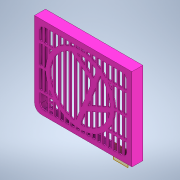
# Autodesk Inventor part: Rambo Case Lid
Saved by Autodesk Inventor 2023 (Build 270158000, 158)
## iProperties
Created: 2019-12-31
Part Number: Rambo Case Lid
Material: Generic
Document SubType Name: Modeling
Designer: pepd9
Density: 1 g/cm^3
Appearance: Default
Author: pepd9
Autodesk Inventor part; units mm, degrees
(part 1 of 2)
ref_plane "YZ Plane" through (0, 0, 0) normal (1, 0, 0) x (0, 1, 0)
ref_plane "XZ Plane" through (0, 0, 0) normal (0, 1, 0) x (-1, 0, 0)
sketch "Sketch1" plane through (0, 0, 0) normal (0, 0, 1) x (1, 0, 0)
  line L0 (3, 53.125) -> (3, 56.125)
  line L1 (3, 56.125) -> (137.52, 56.125)
  line L2 (143.52, 56.125) -> (143.52, 62.125)
  line L3 (143.52, 62.125) -> (-3, 62.125)
  line L4 (-3, 62.125) -> (-3, 53.125)
  line L5 (137.52, -56.125) -> (137.52, 56.125)
  line L6 (143.52, 56.125) -> (143.52, -56.125)
  line L7 (-3, 35.125) -> (-3, 53.125)
  line L8 (143.52, 62.125) -> (-3, 62.125)
  line L9 (-3, 62.125) -> (-3, 53.125)
  line L10 (3, 56.125) -> (33.535898, 56.125)
  line L11 (143.52, 56.125) -> (143.52, 62.125)
  line L12 (-3, 35.125) -> (-3, -52.125)
  arc A0 (-3, -52.125) -> (7, -62.125) centre (7, -52.125) ccw
  line L13 (7, -62.125) -> (143.52, -62.125)
  line L14 (143.52, -62.125) -> (143.52, -56.125)
  line L15 (137.52, -56.125) -> (8, -56.125)
  arc A1 (3, -51.125) -> (8, -56.125) centre (8, -51.125) ccw
  line L16 (3, -51.125) -> (3, 53.125)
  point P0 (0, 0)
  dimension "d0" = 6
  constraints: 34 end point, 4 point on circle, 2 centre point, 1 point on line
  measures "d0" distance between parallel lines of L6 L5
extrude "Extrusion1" add sketch "Sketch1" along normal blind 15
sketch "Sketch2" plane through (0, 0, 15) normal (0, 0, 1) x (1, 0, 0)
  line L0 (-3, 62.125) -> (-3, -52.125) projected
  arc A0 (-3, -52.125) -> (7, -62.125) centre (7, -52.125) ccw projected
  line L1 (7, -62.125) -> (143.52, -62.125) projected
  line L2 (143.52, -62.125) -> (143.52, 62.125) projected
  line L3 (143.52, 62.125) -> (-3, 62.125) projected
  point P0 (0, 0)
extrude "Extrusion2" add sketch "Sketch2" along normal blind 1.5
sketch "Sketch3" plane through (0, 0, 16.5) normal (0, 0, 1) x (1, 0, 0)
  line L0 (5, -47.125) -> (5, 47.125)
  line L1 (12, 54.125) -> (128.52, 54.125)
  line L2 (135.52, 47.125) -> (135.52, -47.125)
  line L3 (128.52, -54.125) -> (12, -54.125)
  arc A0 (5, -47.125) -> (12, -54.125) centre (12, -47.125) ccw
  arc A1 (128.52, -54.125) -> (135.52, -47.125) centre (128.52, -47.125) ccw
  arc A2 (135.52, 47.125) -> (128.52, 54.125) centre (128.52, 47.125) ccw
  arc A3 (12, 54.125) -> (5, 47.125) centre (12, 47.125) ccw
  line L4 (72.76, 54.125) -> (67.76, 54.125)
  line L5 (67.76, 54.125) -> (67.76, -54.125)
  line L6 (67.76, -54.125) -> (72.76, -54.125)
  line L7 (72.76, -54.125) -> (72.76, 54.125)
  line L8 (72.76, 54.125) -> (67.76, -54.125) construction
  line L9 (67.76, 54.125) -> (72.76, -54.125) construction
  line L10 (75.76, 54.125) -> (75.76, -54.125)
  line L11 (75.76, 54.125) -> (80.76, -54.125) construction
  line L12 (80.76, 54.125) -> (75.76, -54.125) construction
  line L13 (80.76, -54.125) -> (80.76, 54.125)
  line L14 (83.76, 54.125) -> (83.76, -54.125)
  line L15 (83.76, 54.125) -> (88.76, -54.125) construction
  line L16 (88.76, 54.125) -> (83.76, -54.125) construction
  line L17 (88.76, -54.125) -> (88.76, 54.125)
  line L18 (91.76, 54.125) -> (91.76, -54.125)
  line L19 (91.76, 54.125) -> (96.76, -54.125) construction
  line L20 (96.76, 54.125) -> (91.76, -54.125) construction
  line L21 (96.76, -54.125) -> (96.76, 54.125)
  line L22 (99.76, 54.125) -> (99.76, -54.125)
  line L23 (99.76, 54.125) -> (104.76, -54.125) construction
  line L24 (104.76, 54.125) -> (99.76, -54.125) construction
  line L25 (104.76, -54.125) -> (104.76, 54.125)
  line L26 (107.76, 54.125) -> (107.76, -54.125)
  line L27 (107.76, 54.125) -> (112.76, -54.125) construction
  line L28 (112.76, 54.125) -> (107.76, -54.125) construction
  line L29 (112.76, -54.125) -> (112.76, 54.125)
  line L30 (115.76, 54.125) -> (115.76, -54.125)
  line L31 (115.76, 54.125) -> (120.76, -54.125) construction
  line L32 (120.76, 54.125) -> (115.76, -54.125) construction
  line L33 (120.76, -54.125) -> (120.76, 54.125)
  line L34 (123.76, 54.125) -> (123.76, -54.125)
  line L35 (123.76, 54.125) -> (128.76, -54.125) construction
  line L36 (128.76, 54.125) -> (123.76, -54.125) construction
  line L37 (128.76, -54.125) -> (128.76, 54.125)
  line L38 (131.76, 54.125) -> (131.76, -54.125)
  line L39 (131.76, 54.125) -> (136.76, -54.125) construction
  line L40 (136.76, 54.125) -> (131.76, -54.125) construction
  line L41 (136.76, -54.125) -> (136.76, 54.125)
  line L42 (59.76, -54.125) -> (64.76, -54.125)
  line L43 (64.76, -54.125) -> (64.76, 54.125)
  line L44 (64.76, 54.125) -> (59.76, 54.125)
  line L45 (59.76, 54.125) -> (59.76, -54.125)
  line L46 (59.76, 54.125) -> (64.76, -54.125) construction
  line L47 (64.76, 54.125) -> (59.76, -54.125) construction
  line L48 (51.76, -54.125) -> (56.76, -54.125)
  line L49 (56.76, -54.125) -> (56.76, 54.125)
  line L50 (56.76, 54.125) -> (51.76, 54.125)
  line L51 (51.76, 54.125) -> (51.76, -54.125)
  line L52 (51.76, 54.125) -> (56.76, -54.125) construction
  line L53 (56.76, 54.125) -> (51.76, -54.125) construction
  line L54 (43.76, -54.125) -> (48.76, -54.125)
  line L55 (48.76, -54.125) -> (48.76, 54.125)
  line L56 (48.76, 54.125) -> (43.76, 54.125)
  line L57 (43.76, 54.125) -> (43.76, -54.125)
  line L58 (43.76, 54.125) -> (48.76, -54.125) construction
  line L59 (48.76, 54.125) -> (43.76, -54.125) construction
  line L60 (35.76, -54.125) -> (40.76, -54.125)
  line L61 (40.76, -54.125) -> (40.76, 54.125)
  line L62 (40.76, 54.125) -> (35.76, 54.125)
  line L63 (35.76, 54.125) -> (35.76, -54.125)
  line L64 (35.76, 54.125) -> (40.76, -54.125) construction
  line L65 (40.76, 54.125) -> (35.76, -54.125) construction
  line L66 (27.76, -54.125) -> (32.76, -54.125)
  line L67 (32.76, -54.125) -> (32.76, 54.125)
  line L68 (32.76, 54.125) -> (27.76, 54.125)
  line L69 (27.76, 54.125) -> (27.76, -54.125)
  line L70 (27.76, 54.125) -> (32.76, -54.125) construction
  line L71 (32.76, 54.125) -> (27.76, -54.125) construction
  line L72 (19.76, -54.125) -> (24.76, -54.125)
  line L73 (24.76, -54.125) -> (24.76, 54.125)
  line L74 (24.76, 54.125) -> (19.76, 54.125)
  line L75 (19.76, 54.125) -> (19.76, -54.125)
  line L76 (19.76, 54.125) -> (24.76, -54.125) construction
  line L77 (24.76, 54.125) -> (19.76, -54.125) construction
  line L78 (11.76, -54.125) -> (16.76, -54.125)
  line L79 (16.76, -54.125) -> (16.76, 54.125)
  line L80 (16.76, 54.125) -> (11.76, 54.125)
  line L81 (11.76, 54.125) -> (11.76, -54.125)
  line L82 (11.76, 54.125) -> (16.76, -54.125) construction
  line L83 (16.76, 54.125) -> (11.76, -54.125) construction
  line L84 (3.76, -54.125) -> (8.76, -54.125)
  line L85 (8.76, -54.125) -> (8.76, 54.125)
  line L86 (8.76, 54.125) -> (3.76, 54.125)
  line L87 (3.76, 54.125) -> (3.76, -54.125)
  line L88 (3.76, 54.125) -> (8.76, -54.125) construction
  line L89 (8.76, 54.125) -> (3.76, -54.125) construction
  line L90 (-3, 62.125) -> (-3, -52.125) projected
  arc A4 (-3, -52.125) -> (7, -62.125) centre (7, -52.125) ccw projected
  line L91 (7, -62.125) -> (143.52, -62.125) projected
  line L92 (143.52, -62.125) -> (143.52, 62.125) projected
  line L93 (143.52, 62.125) -> (-3, 62.125) projected
  point P0 (0, 0)
  point P1 (70.26, 0)
  point P2 (78.26, 0)
  point P3 (86.26, 0)
  point P4 (94.26, 0)
  point P5 (102.26, 0)
  point P6 (110.26, 0)
  point P7 (118.26, 0)
  point P8 (126.26, 0)
  point P9 (134.26, 0)
  point P10 (62.26, 0)
  point P11 (54.26, 0)
  point P12 (46.26, 0)
  point P13 (38.26, 0)
  point P14 (30.26, 0)
  point P15 (22.26, 0)
  point P16 (14.26, 0)
  point P17 (6.26, 0)
  point P18 (8.76, -53.33003)
  point P19 (8.76, 53.33003)
  point P20 (11.76, 54.120885)
  point P21 (11.76, -54.120885)
  point P22 (128.76, -54.120885)
  point P23 (128.76, 54.120885)
  point P24 (131.76, 53.33003)
  point P25 (131.76, -53.33003)
  dimension "d6" = 7
  dimension "d29" = 7
  dimension "d30" = 5
  dimension "d33" = 8
  dimension "d40" = 8
  constraints: 176 end point, 34 midpoint, 8 point on circle, 4 centre point, 4 tangent, 3 horizontal, 2 equal radius, 2 parallel, 1 collinear, 1 perpendicular, 170 other
  measures "d6" radius of A0
  measures "d29" radius of A1
  measures "d30" distance of L6.end L5.end
  measures "d33" distance of L4.end L10.start
  measures "d40" distance of L5.end L42.start
ref_plane "Work Plane1" through (-3, -62.125, 0) normal (0, 0, 1) x (1, 0, 0)
extrude "Extrusion4" cut sketch "Sketch3" against normal through all contours L0 A3 L85 A0 | L81 A3 L1 L79 L3 A0 | L75 L1 L73 L3 | L69 L1 L67 L3 | L63 L1 L61 L3 | L57 L1 L55 L3 | L51 L1 L49 L3 | L45 L1 L43 L3 | L5 L1 L7 L3 | L10 L1 L13 L3 | L14 L1 L17 L3 | L18 L1 L21 L3 | L22 L1 L25 L3 | L26 L1 L29 L3 | L30 L1 L33 L3 | L34 L1 A2 L37 A1 L3 | L38 A2 L2 A1
sketch "Sketch8" plane through (0, 0, 16.5) normal (0, 0, 1) x (1, 0, 0)
  circle A0 centre (65.9053, 0) radius 45
  line L0 (67.76, -54.125) -> (67.76, 54.125)
  line L1 (72.76, -54.125) -> (67.76, -54.125)
  circle A1 centre (65.9053, 0) radius 52
  line L2 (66.135277, -44.999412) -> (96.47099, 33.026332)
  line L3 (58.8415, -44.442128) -> (90.71627, 37.542186)
  line L4 (77.895632, -14.750892) -> (110.904226, -0.31086)
  line L5 (74.316291, -23.957225) -> (110.135552, -8.287631)
  line L6 (83.222966, 18.268842) -> (52.72419, 43.026252)
  line L7 (85.887401, 25.121972) -> (61.648183, 44.79818)
  point P0 (0, 0)
  point P1 (67.76, -44.961763)
  point P2 (67.76, -21.503073)
  point P3 (67.76, -40.820501)
  dimension "d56" = 90
  dimension "d58" = 54.125
  dimension "d59" = 7
  dimension "d60" = 7
  dimension "d61" = 7
  dimension "d62" = 7
  constraints: 12 end point, 4 point on line, 3 parallel, 1 centre point, 10 other
  measures "d58" distance from line of L1 A1.centre
  measures "d60" distance between parallel lines of L2 L3
  measures "d61" distance between parallel lines of L4 L5
  measures "d62" distance between parallel lines of L6 L7
extrude "Extrusion6" add sketch "Sketch8" against normal up to surface (1.5 mm away) contours A0 L0 A1 | L2 L0 L3 A0 | A0 L5 L2 L4 | A0 L0 A1 | L3 L6 L0 L7 | L7 L0 L6 A0 | L2 A0 L3 L0
sketch "Sketch9" plane through (0, 0, 16.5) normal (0, 0, 1) x (1, 0, 0)
  line L0 (83.76, -12.185449) -> (83.76, 0.332706)
  line L1 (83.76, 0.332706) -> (88.76, 13.193084)
  line L2 (88.76, 13.193084) -> (88.76, -9.998135)
  line L3 (88.76, -9.998135) -> (83.76, -12.185449)
  line L4 (80.76, -21.138342) -> (80.76, -42.477499)
  arc A0 (75.76, -43.907686) -> (80.76, -42.477499) centre (65.9053, 0) ccw
  line L5 (75.76, -43.907686) -> (75.76, -23.325656)
  line L6 (75.76, -23.325656) -> (80.76, -21.138342)
  line L7 (91.76, -8.685747) -> (91.76, 20.90931)
  line L8 (91.76, 20.90931) -> (96.47099, 33.026332)
  arc A1 (96.76, 32.756488) -> (96.47099, 33.026332) centre (65.9053, 0) ccw
  line L9 (96.76, 32.756488) -> (96.76, -6.498433)
  line L10 (96.76, -6.498433) -> (91.76, -8.685747)
  line L11 (107.76, -1.686342) -> (107.76, 16.528281)
  arc A2 (110.904226, -0.31086) -> (107.76, 16.528281) centre (65.9053, 0) ccw
  line L12 (110.904226, -0.31086) -> (107.76, -1.686342)
  line L13 (104.76, -10.639235) -> (104.76, -22.700491)
  arc A3 (99.76, -29.645561) -> (104.76, -22.700491) centre (65.9053, 0) ccw
  line L14 (99.76, -29.645561) -> (99.76, -12.826549)
  line L15 (99.76, -12.826549) -> (104.76, -10.639235)
  line L16 (75.76, -0.926469) -> (75.76, 24.326911)
  line L17 (75.76, 24.326911) -> (80.76, 20.268157)
  line L18 (80.76, 20.268157) -> (80.76, 11.933908)
  line L19 (80.76, 11.933908) -> (75.76, -0.926469)
  line L20 (72.76, -27.960124) -> (72.76, -44.474859)
  arc A4 (67.76, -44.961763) -> (72.76, -44.474859) centre (65.9053, 0) ccw
  line L21 (67.76, -44.961763) -> (67.76, -40.820501)
  line L22 (67.76, -40.820501) -> (72.76, -27.960124)
  line L23 (19.76, 23.971051) -> (19.76, 54.125)
  line L24 (19.76, 54.125) -> (24.76, 54.125)
  line L25 (24.76, 54.125) -> (24.76, 31.797237)
  arc A5 (24.76, 31.797237) -> (19.76, 23.971051) centre (65.9053, 0) ccw
  line L26 (51.76, -42.718971) -> (51.76, 42.718971)
  arc A6 (52.72419, 43.026252) -> (51.76, 42.718971) centre (65.9053, 0) ccw
  line L27 (52.72419, 43.026252) -> (56.76, 39.750179)
  line L28 (56.76, 39.750179) -> (56.76, -44.060907)
  arc A7 (51.76, -42.718971) -> (56.76, -44.060907) centre (65.9053, 0) ccw
  line L29 (48.76, -49.092145) -> (48.76, -54.125)
  line L30 (48.76, -54.125) -> (43.76, -54.125)
  line L31 (43.76, -54.125) -> (43.76, -47.048759)
  arc A8 (43.76, -47.048759) -> (48.76, -49.092145) centre (65.9053, 0) ccw
  line L32 (51.76, 50.03909) -> (51.76, 54.125)
  line L33 (51.76, 54.125) -> (56.76, 54.125)
  line L34 (56.76, 54.125) -> (56.76, 51.189486)
  arc A9 (56.76, 51.189486) -> (51.76, 50.03909) centre (65.9053, 0) ccw
  arc A10 (43.76, -39.173788) -> (48.76, -41.605753) centre (65.9053, 0) ccw
  line L35 (43.76, -39.173788) -> (43.76, 39.173788)
  arc A11 (48.76, 41.605753) -> (43.76, 39.173788) centre (65.9053, 0) ccw
  line L36 (48.76, 41.605753) -> (48.76, -41.605753)
  line L37 (112.76, -22.552984) -> (112.76, -54.125)
  line L38 (112.76, -54.125) -> (107.76, -54.125)
  line L39 (107.76, -54.125) -> (107.76, -30.85748)
  arc A12 (107.76, -30.85748) -> (112.76, -22.552984) centre (65.9053, 0) ccw
  line L40 (59.76, -42.079676) -> (59.76, 37.314927)
  line L41 (59.76, 37.314927) -> (64.76, 33.256172)
  line L42 (64.76, 33.256172) -> (64.76, -29.219299)
  line L43 (64.76, -29.219299) -> (59.76, -42.079676)
  arc A13 (19.76, -23.971051) -> (24.76, -31.797237) centre (65.9053, 0) ccw
  line L44 (24.76, -31.797237) -> (24.76, -54.125)
  line L45 (24.76, -54.125) -> (19.76, -54.125)
  line L46 (19.76, -54.125) -> (19.76, -23.971051)
  line L47 (27.76, -23.873334) -> (27.76, 23.873334)
  arc A14 (32.76, 30.436641) -> (27.76, 23.873334) centre (65.9053, 0) ccw
  line L48 (32.76, 30.436641) -> (32.76, -30.436641)
  arc A15 (27.76, -23.873334) -> (32.76, -30.436641) centre (65.9053, 0) ccw
  line L49 (27.76, 35.34029) -> (27.76, 54.125)
  line L50 (27.76, 54.125) -> (32.76, 54.125)
  line L51 (32.76, 54.125) -> (32.76, 40.067307)
  arc A16 (32.76, 40.067307) -> (27.76, 35.34029) centre (65.9053, 0) ccw
  line L52 (35.76, -33.410491) -> (35.76, 33.410491)
  arc A17 (40.76, 37.319082) -> (35.76, 33.410491) centre (65.9053, 0) ccw
  line L53 (40.76, 37.319082) -> (40.76, -37.319082)
  arc A18 (35.76, -33.410491) -> (40.76, -37.319082) centre (65.9053, 0) ccw
  line L54 (35.76, 42.370519) -> (35.76, 54.125)
  line L55 (35.76, 54.125) -> (40.76, 54.125)
  line L56 (40.76, 54.125) -> (40.76, 45.516084)
  arc A19 (40.76, 45.516084) -> (35.76, 42.370519) centre (65.9053, 0) ccw
  line L57 (83.76, -19.825953) -> (88.76, -17.63864)
  line L58 (88.76, -17.63864) -> (88.76, -38.764193)
  arc A20 (83.76, -41.306291) -> (88.76, -38.764193) centre (65.9053, 0) ccw
  line L59 (83.76, -41.306291) -> (83.76, -19.825953)
  line L60 (80.76, -49.8331) -> (80.76, -54.125)
  line L61 (80.76, -54.125) -> (75.76, -54.125)
  line L62 (75.76, -54.125) -> (75.76, -51.057662)
  arc A21 (75.76, -51.057662) -> (80.76, -49.8331) centre (65.9053, 0) ccw
  line L63 (91.76, -16.326251) -> (96.76, -14.138937)
  line L64 (96.76, -14.138937) -> (96.76, -32.756488)
  arc A22 (91.76, -36.831162) -> (96.76, -32.756488) centre (65.9053, 0) ccw
  line L65 (91.76, -36.831162) -> (91.76, -16.326251)
  line L66 (72.76, -51.546223) -> (72.76, -54.125)
  line L67 (72.76, -54.125) -> (67.76, -54.125)
  line L68 (67.76, -54.125) -> (67.76, -51.966913)
  arc A23 (67.76, -51.966913) -> (72.76, -51.546223) centre (65.9053, 0) ccw
  line L69 (107.76, -9.326846) -> (110.135552, -8.287631)
  arc A24 (107.76, -16.528281) -> (110.135552, -8.287631) centre (65.9053, 0) ccw
  line L70 (107.76, -16.528281) -> (107.76, -9.326846)
  line L71 (104.76, -34.558823) -> (104.76, -54.125)
  line L72 (104.76, -54.125) -> (99.76, -54.125)
  line L73 (99.76, -54.125) -> (99.76, -39.469726)
  arc A25 (99.76, -39.469726) -> (104.76, -34.558823) centre (65.9053, 0) ccw
  line L74 (91.76, 45.116898) -> (91.76, 54.125)
  line L75 (91.76, 54.125) -> (96.76, 54.125)
  line L76 (96.76, 54.125) -> (96.76, 41.85675)
  arc A26 (96.76, 41.85675) -> (91.76, 45.116898) centre (65.9053, 0) ccw
  arc A27 (83.76, -48.838609) -> (88.76, -46.708272) centre (65.9053, 0) ccw
  line L77 (88.76, -46.708272) -> (88.76, -54.125)
  line L78 (88.76, -54.125) -> (83.76, -54.125)
  line L79 (83.76, -54.125) -> (83.76, -48.838609)
  line L80 (88.76, 32.510512) -> (85.887401, 25.121972)
  line L81 (85.887401, 25.121972) -> (83.76, 26.848892)
  line L82 (83.76, 26.848892) -> (83.76, 41.306291)
  arc A28 (88.76, 38.764193) -> (83.76, 41.306291) centre (65.9053, 0) ccw
  line L83 (88.76, 38.764193) -> (88.76, 32.510512)
  line L84 (80.76, 42.477499) -> (80.76, 29.284145)
  line L85 (80.76, 29.284145) -> (75.76, 33.342899)
  line L86 (75.76, 33.342899) -> (75.76, 43.907686)
  arc A29 (80.76, 42.477499) -> (75.76, 43.907686) centre (65.9053, 0) ccw
  line L87 (72.76, 44.474859) -> (72.76, 35.778152)
  line L88 (72.76, 35.778152) -> (67.76, 39.836907)
  line L89 (67.76, 39.836907) -> (67.76, 44.961763)
  arc A30 (72.76, 44.474859) -> (67.76, 44.961763) centre (65.9053, 0) ccw
  line L90 (64.76, 44.985423) -> (64.76, 42.27216)
  line L91 (64.76, 42.27216) -> (61.648183, 44.79818)
  arc A31 (64.76, 44.985423) -> (61.648183, 44.79818) centre (65.9053, 0) ccw
  line L92 (104.76, -2.99873) -> (99.76, -5.186044)
  line L93 (99.76, -5.186044) -> (99.76, 29.645561)
  arc A32 (104.76, 22.700491) -> (99.76, 29.645561) centre (65.9053, 0) ccw
  line L94 (104.76, 22.700491) -> (104.76, -2.99873)
  line L95 (80.76, -13.497837) -> (77.895632, -14.750892)
  line L96 (77.895632, -14.750892) -> (80.76, -7.38352)
  line L97 (80.76, -7.38352) -> (80.76, -13.497837)
  arc A33 (64.76, 51.987386) -> (59.76, 51.635601) centre (65.9053, 0) ccw
  line L98 (59.76, 51.635601) -> (59.76, 54.125)
  line L99 (59.76, 54.125) -> (64.76, 54.125)
  line L100 (64.76, 54.125) -> (64.76, 51.987386)
  line L101 (72.76, -8.642695) -> (67.76, -21.503073)
  line L102 (67.76, -21.503073) -> (67.76, 30.820919)
  line L103 (67.76, 30.820919) -> (72.76, 26.762164)
  line L104 (72.76, 26.762164) -> (72.76, -8.642695)
  arc A34 (80.76, 49.8331) -> (75.76, 51.057662) centre (65.9053, 0) ccw
  line L105 (75.76, 51.057662) -> (75.76, 54.125)
  line L106 (75.76, 54.125) -> (80.76, 54.125)
  line L107 (80.76, 54.125) -> (80.76, 49.8331)
  arc A35 (88.76, 46.708272) -> (83.76, 48.838609) centre (65.9053, 0) ccw
  line L108 (83.76, 48.838609) -> (83.76, 54.125)
  line L109 (83.76, 54.125) -> (88.76, 54.125)
  line L110 (88.76, 54.125) -> (88.76, 46.708272)
  arc A36 (104.76, 34.558823) -> (99.76, 39.469726) centre (65.9053, 0) ccw
  line L111 (99.76, 39.469726) -> (99.76, 54.125)
  line L112 (99.76, 54.125) -> (104.76, 54.125)
  line L113 (104.76, 54.125) -> (104.76, 34.558823)
  arc A37 (91.76, -45.116898) -> (96.76, -41.85675) centre (65.9053, 0) ccw
  line L114 (96.76, -41.85675) -> (96.76, -54.125)
  line L115 (96.76, -54.125) -> (91.76, -54.125)
  line L116 (91.76, -54.125) -> (91.76, -45.116898)
  arc A38 (72.76, 51.546223) -> (67.76, 51.966913) centre (65.9053, 0) ccw
  line L117 (67.76, 51.966913) -> (67.76, 54.125)
  line L118 (67.76, 54.125) -> (72.76, 54.125)
  line L119 (72.76, 54.125) -> (72.76, 51.546223)
  line L120 (16.76, -16.992336) -> (16.76, -54.125)
  line L121 (16.76, -54.125) -> (12, -54.125)
  arc A39 (11.76, -54.120885) -> (12, -54.125) centre (12, -47.125) ccw
  line L122 (11.76, -54.120885) -> (11.76, 54.120885)
  arc A40 (12, 54.125) -> (11.76, 54.120885) centre (12, 47.125) ccw
  line L123 (12, 54.125) -> (16.76, 54.125)
  line L124 (16.76, 54.125) -> (16.76, 16.992336)
  arc A41 (16.76, 16.992336) -> (16.76, -16.992336) centre (65.9053, 0) ccw
  arc A42 (51.76, -50.03909) -> (56.76, -51.189486) centre (65.9053, 0) ccw
  line L125 (56.76, -51.189486) -> (56.76, -54.125)
  line L126 (56.76, -54.125) -> (51.76, -54.125)
  line L127 (51.76, -54.125) -> (51.76, -50.03909)
  arc A43 (24.76, 18.222631) -> (24.76, -18.222631) centre (65.9053, 0) ccw
  line L128 (24.76, 18.222631) -> (24.76, -18.222631)
  arc A44 (35.76, -42.370519) -> (40.76, -45.516084) centre (65.9053, 0) ccw
  line L129 (40.76, -45.516084) -> (40.76, -54.125)
  line L130 (40.76, -54.125) -> (35.76, -54.125)
  line L131 (35.76, -54.125) -> (35.76, -42.370519)
  line L132 (115.76, 14.782046) -> (115.76, 54.125)
  line L133 (115.76, 54.125) -> (120.76, 54.125)
  line L134 (120.76, 54.125) -> (120.76, -54.125)
  line L135 (120.76, -54.125) -> (115.76, -54.125)
  line L136 (115.76, -54.125) -> (115.76, -14.782046)
  arc A45 (115.76, -14.782046) -> (115.76, 14.782046) centre (65.9053, 0) ccw
  line L137 (-3, 62.125) -> (-3, -52.125)
  arc A46 (-3, -52.125) -> (7, -62.125) centre (7, -52.125) ccw
  line L138 (7, -62.125) -> (143.52, -62.125)
  arc A47 (131.76, -53.33003) -> (135.52, -47.125) centre (128.52, -47.125) ccw
  line L139 (131.76, -53.33003) -> (131.76, 53.33003)
  arc A48 (135.52, 47.125) -> (131.76, 53.33003) centre (128.52, 47.125) ccw
  line L140 (135.52, 47.125) -> (135.52, -47.125)
  line L141 (5, -47.125) -> (5, 47.125)
  arc A49 (8.76, 53.33003) -> (5, 47.125) centre (12, 47.125) ccw
  line L142 (8.76, 53.33003) -> (8.76, -53.33003)
  arc A50 (5, -47.125) -> (8.76, -53.33003) centre (12, -47.125) ccw
  line L143 (123.76, 54.125) -> (128.52, 54.125)
  arc A51 (128.76, 54.120885) -> (128.52, 54.125) centre (128.52, 47.125) ccw
  line L144 (128.76, 54.120885) -> (128.76, -54.120885)
  arc A52 (128.52, -54.125) -> (128.76, -54.120885) centre (128.52, -47.125) ccw
  line L145 (128.52, -54.125) -> (123.76, -54.125)
  line L146 (123.76, -54.125) -> (123.76, 54.125)
  arc A53 (27.76, -35.34029) -> (32.76, -40.067307) centre (65.9053, 0) ccw
  line L147 (32.76, -40.067307) -> (32.76, -54.125)
  line L148 (32.76, -54.125) -> (27.76, -54.125)
  line L149 (27.76, -54.125) -> (27.76, -35.34029)
  arc A54 (59.76, -51.635601) -> (64.76, -51.987386) centre (65.9053, 0) ccw
  line L150 (64.76, -51.987386) -> (64.76, -54.125)
  line L151 (64.76, -54.125) -> (59.76, -54.125)
  line L152 (59.76, -54.125) -> (59.76, -51.635601)
  arc A55 (112.76, 22.552984) -> (107.76, 30.85748) centre (65.9053, 0) ccw
  line L153 (107.76, 30.85748) -> (107.76, 54.125)
  line L154 (107.76, 54.125) -> (112.76, 54.125)
  line L155 (112.76, 54.125) -> (112.76, 22.552984)
  arc A56 (48.76, 49.092145) -> (43.76, 47.048759) centre (65.9053, 0) ccw
  line L156 (43.76, 47.048759) -> (43.76, 54.125)
  line L157 (43.76, 54.125) -> (48.76, 54.125)
  line L158 (48.76, 54.125) -> (48.76, 49.092145)
  arc A57 (115.76, -14.782046) -> (115.76, 14.782046) centre (65.9053, 0) ccw
  circle A58 centre (65.9053, 0) radius 52
  line L159 (135.52, 47.125) -> (135.52, -47.125)
  line L160 (5, -47.125) -> (5, 47.125)
  line L161 (135.52, -34.125) -> (5, -34.125)
  line L162 (5, -34.125) -> (5, -30.125)
  line L163 (5, -30.125) -> (135.52, -30.125)
  line L164 (135.52, -30.125) -> (135.52, -34.125)
  line L165 (135.52, 30.125) -> (5, 30.125)
  line L166 (5, 30.125) -> (5, 34.125)
  line L167 (5, 34.125) -> (135.52, 34.125)
  line L168 (135.52, 34.125) -> (135.52, 30.125)
  line L169 (143.52, -62.125) -> (143.52, 62.125)
  line L170 (143.52, 62.125) -> (-3, 62.125)
  point P0 (0, 0)
  point P1 (8.76, 34.125)
  point P2 (5, 30.125)
  point P3 (8.76, 30.125)
  point P4 (16.76, 34.125)
  point P5 (11.76, 34.125)
  point P6 (11.76, 30.125)
  point P7 (16.76, 30.125)
  point P8 (24.76, 34.125)
  point P9 (19.76, 34.125)
  point P10 (19.76, 30.125)
  point P11 (23.520345, 30.125)
  point P12 (8.76, -30.125)
  point P13 (5, -34.125)
  point P14 (8.76, -34.125)
  point P15 (16.76, -30.125)
  point P16 (11.76, -30.125)
  point P17 (11.76, -34.125)
  point P18 (16.76, -34.125)
  point P19 (23.520345, -30.125)
  point P20 (19.76, -30.125)
  point P21 (19.76, -34.125)
  point P22 (24.76, -34.125)
  point P23 (112.76, 34.125)
  point P24 (107.76, 34.125)
  point P25 (108.290254, 30.125)
  point P26 (112.76, 30.125)
  point P27 (120.76, 34.125)
  point P28 (115.76, 34.125)
  point P29 (115.76, 30.125)
  point P30 (120.76, 30.125)
  point P31 (128.76, 34.125)
  point P32 (123.76, 34.125)
  point P33 (123.76, 30.125)
  point P34 (128.76, 30.125)
  point P35 (131.76, 34.125)
  point P36 (131.76, 30.125)
  point P37 (112.76, -30.125)
  point P38 (108.290254, -30.125)
  point P39 (107.76, -34.125)
  point P40 (112.76, -34.125)
  point P41 (120.76, -30.125)
  point P42 (115.76, -30.125)
  point P43 (115.76, -34.125)
  point P44 (120.76, -34.125)
  point P45 (128.76, -30.125)
  point P46 (123.76, -30.125)
  point P47 (123.76, -34.125)
  point P48 (128.76, -34.125)
  point P49 (131.76, -30.125)
  point P50 (131.76, -34.125)
  dimension "d65" = 4
  dimension "d66" = 4
  dimension "d67" = 20
  dimension "d68" = 20
  constraints: 16 end point, 4 parallel, 4 point on line, 2 horizontal, 2 perpendicular, 1 coincident, 3 other
  measures "d65" distance of L161.end L162.end
  measures "d66" distance of L165.end L166.end
  measures "d67" distance from line of L44.end L161
  measures "d68" distance from line of L123.end L167
extrude "Extrusion7" add sketch "Sketch9" against normal up to surface (1.5 mm away) contours L163 L37 L161 L39 A12 | L163 L134 L161 L136 | L165 L132 L167 L134 | L163 L144 L161 L146 | L146 L167 L144 L165 | L165 A55 L153 L167 L155 | L163 L140 L161 L139 | L139 L167 L140 L165 | L44 L161 L46 L163 A13 | A5 L165 L23 L167 L25 | L161 L122 L163 L120 | L124 L165 L122 L167 | L161 L141 L163 L142 | L142 L165 L141 L167
sketch "Sketch10" plane through (0, 0, 16.5) normal (0, 0, 1) x (1, 0, 0)
  line L0 (135.52, -30.125) -> (135.52, 30.125)
  line L1 (5, 30.125) -> (5, -30.125)
  line L2 (135.52, -2) -> (5, -2)
  line L3 (5, -2) -> (5, 2)
  line L4 (5, 2) -> (135.52, 2)
  line L5 (135.52, 2) -> (135.52, -2)
  line L6 (5, 30.125) -> (5, -30.125)
  arc A0 (115.76, -14.782046) -> (115.76, 14.782046) centre (65.9053, 0) ccw
  arc A1 (16.76, 16.992336) -> (16.76, -16.992336) centre (65.9053, 0) ccw
  point P0 (0, 0)
  point P1 (5, 2.125)
  point P2 (5, 0)
  point P3 (13.943776, -2)
  point P4 (13.943776, 2)
  point P5 (117.866824, 2)
  point P6 (117.866824, -2)
  dimension "d71" = 2
  dimension "d72" = 2
  constraints: 8 end point, 2 parallel, 2 point on line, 1 horizontal, 1 midpoint, 1 perpendicular
  measures "d71" distance from line of L2 point (5, 0)
  measures "d72" distance from line of point (5, 0) L4
extrude "Extrusion8" add sketch "Sketch10" against normal up to surface (1.5 mm away) contours L2 A0 L4 L0 | L2 L1 L4 A1
ref_plane "Work Plane2" through (123.52, -58.125, 13.5) normal (0, 0, 1) x (1, 0, 0)
ref_plane "Work Plane3" through (123.52, -58.125, 13) normal (0, 0, 1) x (1, 0, 0)
fillet "Fillet1" radius 0.4 25 edges at (131.76, -53.33, 15.75) (131.76, -34.125, 15.75) (135.52, -34.125, 15.75) (128.76, -34.125, 15.75) (123.76, -34.125, 15.75) (128.76, -54.1209, 15.75) (123.76, -54.125, 15.75) (120.76, -54.125, 15.75) (115.76, -54.125, 15.75) (115.76, -34.125, 15.75) (120.76, -34.125, 15.75) (112.76, -54.125, 15.75) (107.76, -54.125, 15.75) (107.76, -34.125, 15.75) (112.76, -34.125, 15.75) (104.76, -54.125, 15.75) (99.76, -54.125, 15.75) (96.76, -54.125, 15.75) (91.76, -54.125, 15.75) (88.76, -54.125, 15.75) (83.76, -54.125, 15.75) (80.76, -54.125, 15.75) (75.76, -54.125, 15.75) (72.76, -54.125, 15.75) (67.76, -54.125, 15.75)
fillet "Fillet2" radius 0.4 26 edges at (64.76, -54.125, 15.75) (59.76, -54.125, 15.75) (56.76, -54.125, 15.75) (51.76, -54.125, 15.75) (48.76, -54.125, 15.75) (43.76, -54.125, 15.75) (40.76, -54.125, 15.75) (35.76, -54.125, 15.75) (32.76, -54.125, 15.75) (27.76, -54.125, 15.75) (24.76, -54.125, 15.75) (19.76, -54.125, 15.75) (16.76, -54.125, 15.75) (11.76, -54.1209, 15.75) (8.76, -53.33, 15.75) (5, -34.125, 15.75) (8.76, -34.125, 15.75) (11.76, -34.125, 15.75) (16.76, -34.125, 15.75) (19.76, -34.125, 15.75) (24.76, -34.125, 15.75) (5, -30.125, 15.75) (8.76, -30.125, 15.75) (11.76, -30.125, 15.75) (16.76, -30.125, 15.75) (19.76, -30.125, 15.75)
fillet "Fillet3" radius 0.4 25 edges at (11.76, -2, 15.75) (8.76, -2, 15.75) (5, -2, 15.75) (5, 2, 15.75) (8.76, 2, 15.75) (11.76, 2, 15.75) (5, 30.125, 15.75) (8.76, 30.125, 15.75) (11.76, 30.125, 15.75) (16.76, 30.125, 15.75) (16.76, 34.125, 15.75) (11.76, 34.125, 15.75) (8.76, 34.125, 15.75) (5, 34.125, 15.75) (8.76, 53.33, 15.75) (11.76, 54.1209, 15.75) (16.76, 54.125, 15.75) (19.76, 30.125, 15.75) (19.76, 34.125, 15.75) (24.76, 54.125, 15.75) (19.76, 54.125, 15.75) (32.76, 54.125, 15.75) (27.76, 54.125, 15.75) (35.76, 54.125, 15.75) (40.76, 54.125, 15.75)
fillet "Fillet4" radius 0.4 24 edges at (43.76, 54.125, 15.75) (48.76, 54.125, 15.75) (51.76, 54.125, 15.75) (56.76, 54.125, 15.75) (59.76, 54.125, 15.75) (64.76, 54.125, 15.75) (67.76, 54.125, 15.75) (72.76, 54.125, 15.75) (75.76, 54.125, 15.75) (80.76, 54.125, 15.75) (83.76, 54.125, 15.75) (88.76, 54.125, 15.75) (91.76, 54.125, 15.75) (96.76, 54.125, 15.75) (99.76, 54.125, 15.75) (104.76, 54.125, 15.75) (107.76, 54.125, 15.75) (120.76, 54.125, 15.75) (115.76, 54.125, 15.75) (128.76, 54.1209, 15.75) (123.76, 54.125, 15.75) (131.76, 53.33, 15.75) (135.52, 34.125, 15.75) (131.76, 34.125, 15.75)
fillet "Fillet5" radius 0.4 31 edges at (128.76, 34.125, 15.75) (123.76, 34.125, 15.75) (120.76, 34.125, 15.75) (115.76, 34.125, 15.75) (112.76, 30.125, 15.75) (112.76, 34.125, 15.75) (112.76, 54.125, 15.75) (107.76, 34.125, 15.75) (120.76, 30.125, 15.75) (115.76, 30.125, 15.75) (123.76, 30.125, 15.75) (131.76, 30.125, 15.75) (128.76, 30.125, 15.75) (135.52, 30.125, 15.75) (135.52, 2, 15.75) (131.76, 2, 15.75) (128.76, 2, 15.75) (123.76, 2, 15.75) (120.76, 2, 15.75) (120.76, -2, 15.75) (123.76, -2, 15.75) (128.76, -2, 15.75) (131.76, -2, 15.75) (135.52, -2, 15.75) (135.52, -30.125, 15.75) (131.76, -30.125, 15.75) (128.76, -30.125, 15.75) (123.76, -30.125, 15.75) (120.76, -30.125, 15.75) (115.76, -30.125, 15.75) (112.76, -30.125, 15.75)
chamfer "Chamfer1" distance 0.25 angle 45 3 edges at (75.26, -62.125, 16.5) (-3, 5, 16.5) (-0.0711, -59.1961, 16.5)
sketch "Sketch13" plane through (0, 0, 16.5) normal (0, 0, 1) x (1, 0, 0)
  line L0 (143.52, -61.875) -> (7, -61.875)
  line L1 (-2.75, -52.125) -> (-2.75, 62.125)
  arc A0 (-2.75, -52.125) -> (7, -61.875) centre (7, -52.125) ccw
  arc A1 (48.76, 49.092145) -> (43.76, 47.048759) centre (65.9053, 0) ccw
  line L2 (43.76, 47.048759) -> (43.76, 53.725)
  arc A2 (44.16, 54.125) -> (43.76, 53.725) centre (44.16, 53.725) ccw
  line L3 (44.16, 54.125) -> (48.36, 54.125)
  arc A3 (48.76, 53.725) -> (48.36, 54.125) centre (48.36, 53.725) ccw
  line L4 (48.76, 53.725) -> (48.76, 49.092145)
  line L5 (108.290254, 30.125) -> (112.36, 30.125)
  arc A4 (112.76, 29.725) -> (112.36, 30.125) centre (112.36, 29.725) ccw
  line L6 (112.76, 29.725) -> (112.76, 22.552984)
  arc A5 (112.76, 22.552984) -> (108.290254, 30.125) centre (65.9053, 0) ccw
  arc A6 (59.76, -51.635601) -> (64.76, -51.987386) centre (65.9053, 0) ccw
  line L7 (64.76, -51.987386) -> (64.76, -53.725)
  arc A7 (64.36, -54.125) -> (64.76, -53.725) centre (64.36, -53.725) ccw
  line L8 (64.36, -54.125) -> (60.16, -54.125)
  arc A8 (59.76, -53.725) -> (60.16, -54.125) centre (60.16, -53.725) ccw
  line L9 (59.76, -53.725) -> (59.76, -51.635601)
  arc A9 (27.76, -35.34029) -> (32.76, -40.067307) centre (65.9053, 0) ccw
  line L10 (32.76, -40.067307) -> (32.76, -53.725)
  arc A10 (32.36, -54.125) -> (32.76, -53.725) centre (32.36, -53.725) ccw
  line L11 (32.36, -54.125) -> (28.16, -54.125)
  arc A11 (27.76, -53.725) -> (28.16, -54.125) centre (28.16, -53.725) ccw
  line L12 (27.76, -53.725) -> (27.76, -35.34029)
  line L13 (128.36, 34.125) -> (124.16, 34.125)
  arc A12 (123.76, 34.525) -> (124.16, 34.125) centre (124.16, 34.525) ccw
  line L14 (123.76, 34.525) -> (123.76, 53.725)
  arc A13 (124.16, 54.125) -> (123.76, 53.725) centre (124.16, 53.725) ccw
  line L15 (124.16, 54.125) -> (128.36, 54.125)
  arc A14 (128.76, 53.725) -> (128.36, 54.125) centre (128.36, 53.725) ccw
  line L16 (128.76, 53.725) -> (128.76, 34.525)
  arc A15 (128.36, 34.125) -> (128.76, 34.525) centre (128.36, 34.525) ccw
  line L17 (5.4, -34.125) -> (8.36, -34.125)
  arc A16 (8.76, -34.525) -> (8.36, -34.125) centre (8.36, -34.525) ccw
  line L18 (8.76, -34.525) -> (8.76, -52.630488)
  arc A17 (8.139394, -52.964154) -> (8.76, -52.630488) centre (8.36, -52.630488) ccw
  arc A18 (5, -47.125) -> (8.139394, -52.964154) centre (12, -47.125) ccw
  line L19 (5, -47.125) -> (5, -34.525)
  arc A19 (5.4, -34.125) -> (5, -34.525) centre (5.4, -34.525) ccw
  line L20 (135.12, 34.125) -> (132.16, 34.125)
  arc A20 (131.76, 34.525) -> (132.16, 34.125) centre (132.16, 34.525) ccw
  line L21 (131.76, 34.525) -> (131.76, 52.630488)
  arc A21 (132.380606, 52.964154) -> (131.76, 52.630488) centre (132.16, 52.630488) ccw
  arc A22 (135.52, 47.125) -> (132.380606, 52.964154) centre (128.52, 47.125) ccw
  line L22 (135.52, 47.125) -> (135.52, 34.525)
  arc A23 (135.12, 34.125) -> (135.52, 34.525) centre (135.12, 34.525) ccw
  arc A24 (35.76, -42.370519) -> (40.76, -45.516084) centre (65.9053, 0) ccw
  line L23 (40.76, -45.516084) -> (40.76, -53.725)
  arc A25 (40.36, -54.125) -> (40.76, -53.725) centre (40.36, -53.725) ccw
  line L24 (40.36, -54.125) -> (36.16, -54.125)
  arc A26 (35.76, -53.725) -> (36.16, -54.125) centre (36.16, -53.725) ccw
  line L25 (35.76, -53.725) -> (35.76, -42.370519)
  arc A27 (24.76, 18.222631) -> (24.76, -18.222631) centre (65.9053, 0) ccw
  line L26 (24.76, 18.222631) -> (24.76, -18.222631)
  arc A28 (51.76, -50.03909) -> (56.76, -51.189486) centre (65.9053, 0) ccw
  line L27 (56.76, -51.189486) -> (56.76, -53.725)
  arc A29 (56.36, -54.125) -> (56.76, -53.725) centre (56.36, -53.725) ccw
  line L28 (56.36, -54.125) -> (52.16, -54.125)
  arc A30 (51.76, -53.725) -> (52.16, -54.125) centre (52.16, -53.725) ccw
  line L29 (51.76, -53.725) -> (51.76, -50.03909)
  line L30 (12.16, -34.125) -> (16.36, -34.125)
  arc A31 (16.76, -34.525) -> (16.36, -34.125) centre (16.36, -34.525) ccw
  line L31 (16.76, -34.525) -> (16.76, -53.725)
  arc A32 (16.36, -54.125) -> (16.76, -53.725) centre (16.36, -53.725) ccw
  line L32 (16.36, -54.125) -> (12.16, -54.125)
  arc A33 (11.76, -53.725) -> (12.16, -54.125) centre (12.16, -53.725) ccw
  line L33 (11.76, -53.725) -> (11.76, -34.525)
  arc A34 (12.16, -34.125) -> (11.76, -34.525) centre (12.16, -34.525) ccw
  arc A35 (72.76, 51.546223) -> (67.76, 51.966913) centre (65.9053, 0) ccw
  line L34 (67.76, 51.966913) -> (67.76, 53.725)
  arc A36 (68.16, 54.125) -> (67.76, 53.725) centre (68.16, 53.725) ccw
  line L35 (68.16, 54.125) -> (72.36, 54.125)
  arc A37 (72.76, 53.725) -> (72.36, 54.125) centre (72.36, 53.725) ccw
  line L36 (72.76, 53.725) -> (72.76, 51.546223)
  arc A38 (91.76, -45.116898) -> (96.76, -41.85675) centre (65.9053, 0) ccw
  line L37 (96.76, -41.85675) -> (96.76, -53.725)
  arc A39 (96.36, -54.125) -> (96.76, -53.725) centre (96.36, -53.725) ccw
  line L38 (96.36, -54.125) -> (92.16, -54.125)
  arc A40 (91.76, -53.725) -> (92.16, -54.125) centre (92.16, -53.725) ccw
  line L39 (91.76, -53.725) -> (91.76, -45.116898)
  arc A41 (104.76, 34.558823) -> (99.76, 39.469726) centre (65.9053, 0) ccw
  line L40 (99.76, 39.469726) -> (99.76, 53.725)
  arc A42 (100.16, 54.125) -> (99.76, 53.725) centre (100.16, 53.725) ccw
  line L41 (100.16, 54.125) -> (104.36, 54.125)
  arc A43 (104.76, 53.725) -> (104.36, 54.125) centre (104.36, 53.725) ccw
  line L42 (104.76, 53.725) -> (104.76, 34.558823)
  arc A44 (88.76, 46.708272) -> (83.76, 48.838609) centre (65.9053, 0) ccw
  line L43 (83.76, 48.838609) -> (83.76, 53.725)
  arc A45 (84.16, 54.125) -> (83.76, 53.725) centre (84.16, 53.725) ccw
  line L44 (84.16, 54.125) -> (88.36, 54.125)
  arc A46 (88.76, 53.725) -> (88.36, 54.125) centre (88.36, 53.725) ccw
  line L45 (88.76, 53.725) -> (88.76, 46.708272)
  arc A47 (80.76, 49.8331) -> (75.76, 51.057662) centre (65.9053, 0) ccw
  line L46 (75.76, 51.057662) -> (75.76, 53.725)
  arc A48 (76.16, 54.125) -> (75.76, 53.725) centre (76.16, 53.725) ccw
  line L47 (76.16, 54.125) -> (80.36, 54.125)
  arc A49 (80.76, 53.725) -> (80.36, 54.125) centre (80.36, 53.725) ccw
  line L48 (80.76, 53.725) -> (80.76, 49.8331)
  line L49 (72.76, -8.642695) -> (67.76, -21.503073)
  line L50 (67.76, -21.503073) -> (67.76, 30.820919)
  line L51 (67.76, 30.820919) -> (72.76, 26.762164)
  line L52 (72.76, 26.762164) -> (72.76, -8.642695)
  arc A50 (64.76, 51.987386) -> (59.76, 51.635601) centre (65.9053, 0) ccw
  line L53 (59.76, 51.635601) -> (59.76, 53.725)
  arc A51 (60.16, 54.125) -> (59.76, 53.725) centre (60.16, 53.725) ccw
  line L54 (60.16, 54.125) -> (64.36, 54.125)
  arc A52 (64.76, 53.725) -> (64.36, 54.125) centre (64.36, 53.725) ccw
  line L55 (64.76, 53.725) -> (64.76, 51.987386)
  line L56 (80.76, -13.497837) -> (77.895632, -14.750892)
  line L57 (77.895632, -14.750892) -> (80.76, -7.38352)
  line L58 (80.76, -7.38352) -> (80.76, -13.497837)
  line L59 (104.76, -2.99873) -> (99.76, -5.186044)
  line L60 (99.76, -5.186044) -> (99.76, 29.645561)
  arc A53 (104.76, 22.700491) -> (99.76, 29.645561) centre (65.9053, 0) ccw
  line L61 (104.76, 22.700491) -> (104.76, -2.99873)
  line L62 (64.76, 44.985423) -> (64.76, 42.27216)
  line L63 (64.76, 42.27216) -> (61.648183, 44.79818)
  arc A54 (64.76, 44.985423) -> (61.648183, 44.79818) centre (65.9053, 0) ccw
  line L64 (72.76, 44.474859) -> (72.76, 35.778152)
  line L65 (72.76, 35.778152) -> (67.76, 39.836907)
  line L66 (67.76, 39.836907) -> (67.76, 44.961763)
  arc A55 (72.76, 44.474859) -> (67.76, 44.961763) centre (65.9053, 0) ccw
  line L67 (80.76, 42.477499) -> (80.76, 29.284145)
  line L68 (80.76, 29.284145) -> (75.76, 33.342899)
  line L69 (75.76, 33.342899) -> (75.76, 43.907686)
  arc A56 (80.76, 42.477499) -> (75.76, 43.907686) centre (65.9053, 0) ccw
  line L70 (88.76, 32.510512) -> (85.887401, 25.121972)
  line L71 (85.887401, 25.121972) -> (83.76, 26.848892)
  line L72 (83.76, 26.848892) -> (83.76, 41.306291)
  arc A57 (88.76, 38.764193) -> (83.76, 41.306291) centre (65.9053, 0) ccw
  line L73 (88.76, 38.764193) -> (88.76, 32.510512)
  arc A58 (83.76, -48.838609) -> (88.76, -46.708272) centre (65.9053, 0) ccw
  line L74 (88.76, -46.708272) -> (88.76, -53.725)
  arc A59 (88.36, -54.125) -> (88.76, -53.725) centre (88.36, -53.725) ccw
  line L75 (88.36, -54.125) -> (84.16, -54.125)
  arc A60 (83.76, -53.725) -> (84.16, -54.125) centre (84.16, -53.725) ccw
  line L76 (83.76, -53.725) -> (83.76, -48.838609)
  line L77 (91.76, 45.116898) -> (91.76, 53.725)
  arc A61 (92.16, 54.125) -> (91.76, 53.725) centre (92.16, 53.725) ccw
  line L78 (92.16, 54.125) -> (96.36, 54.125)
  arc A62 (96.76, 53.725) -> (96.36, 54.125) centre (96.36, 53.725) ccw
  line L79 (96.76, 53.725) -> (96.76, 41.85675)
  arc A63 (96.76, 41.85675) -> (91.76, 45.116898) centre (65.9053, 0) ccw
  line L80 (104.76, -34.558823) -> (104.76, -53.725)
  arc A64 (104.36, -54.125) -> (104.76, -53.725) centre (104.36, -53.725) ccw
  line L81 (104.36, -54.125) -> (100.16, -54.125)
  arc A65 (99.76, -53.725) -> (100.16, -54.125) centre (100.16, -53.725) ccw
  line L82 (99.76, -53.725) -> (99.76, -39.469726)
  arc A66 (99.76, -39.469726) -> (104.76, -34.558823) centre (65.9053, 0) ccw
  line L83 (107.76, -9.326846) -> (110.135552, -8.287631)
  arc A67 (107.76, -16.528281) -> (110.135552, -8.287631) centre (65.9053, 0) ccw
  line L84 (107.76, -16.528281) -> (107.76, -9.326846)
  line L85 (72.76, -51.546223) -> (72.76, -53.725)
  arc A68 (72.36, -54.125) -> (72.76, -53.725) centre (72.36, -53.725) ccw
  line L86 (72.36, -54.125) -> (68.16, -54.125)
  arc A69 (67.76, -53.725) -> (68.16, -54.125) centre (68.16, -53.725) ccw
  line L87 (67.76, -53.725) -> (67.76, -51.966913)
  arc A70 (67.76, -51.966913) -> (72.76, -51.546223) centre (65.9053, 0) ccw
  line L88 (91.76, -16.326251) -> (96.76, -14.138937)
  line L89 (96.76, -14.138937) -> (96.76, -32.756488)
  arc A71 (91.76, -36.831162) -> (96.76, -32.756488) centre (65.9053, 0) ccw
  line L90 (91.76, -36.831162) -> (91.76, -16.326251)
  line L91 (80.76, -49.8331) -> (80.76, -53.725)
  arc A72 (80.36, -54.125) -> (80.76, -53.725) centre (80.36, -53.725) ccw
  line L92 (80.36, -54.125) -> (76.16, -54.125)
  arc A73 (75.76, -53.725) -> (76.16, -54.125) centre (76.16, -53.725) ccw
  line L93 (75.76, -53.725) -> (75.76, -51.057662)
  arc A74 (75.76, -51.057662) -> (80.76, -49.8331) centre (65.9053, 0) ccw
  line L94 (83.76, -19.825953) -> (88.76, -17.63864)
  line L95 (88.76, -17.63864) -> (88.76, -38.764193)
  arc A75 (83.76, -41.306291) -> (88.76, -38.764193) centre (65.9053, 0) ccw
  line L96 (83.76, -41.306291) -> (83.76, -19.825953)
  line L97 (35.76, 42.370519) -> (35.76, 53.725)
  arc A76 (36.16, 54.125) -> (35.76, 53.725) centre (36.16, 53.725) ccw
  line L98 (36.16, 54.125) -> (40.36, 54.125)
  arc A77 (40.76, 53.725) -> (40.36, 54.125) centre (40.36, 53.725) ccw
  line L99 (40.76, 53.725) -> (40.76, 45.516084)
  arc A78 (40.76, 45.516084) -> (35.76, 42.370519) centre (65.9053, 0) ccw
  line L100 (35.76, -33.410491) -> (35.76, 33.410491)
  arc A79 (40.76, 37.319082) -> (35.76, 33.410491) centre (65.9053, 0) ccw
  line L101 (40.76, 37.319082) -> (40.76, -37.319082)
  arc A80 (35.76, -33.410491) -> (40.76, -37.319082) centre (65.9053, 0) ccw
  line L102 (27.76, 35.34029) -> (27.76, 53.725)
  arc A81 (28.16, 54.125) -> (27.76, 53.725) centre (28.16, 53.725) ccw
  line L103 (28.16, 54.125) -> (32.36, 54.125)
  arc A82 (32.76, 53.725) -> (32.36, 54.125) centre (32.36, 53.725) ccw
  line L104 (32.76, 53.725) -> (32.76, 40.067307)
  arc A83 (32.76, 40.067307) -> (27.76, 35.34029) centre (65.9053, 0) ccw
  line L105 (27.76, -23.873334) -> (27.76, 23.873334)
  arc A84 (32.76, 30.436641) -> (27.76, 23.873334) centre (65.9053, 0) ccw
  line L106 (32.76, 30.436641) -> (32.76, -30.436641)
  arc A85 (27.76, -23.873334) -> (32.76, -30.436641) centre (65.9053, 0) ccw
  line L107 (23.520345, -30.125) -> (20.16, -30.125)
  arc A86 (19.76, -29.725) -> (20.16, -30.125) centre (20.16, -29.725) ccw
  line L108 (19.76, -29.725) -> (19.76, -23.971051)
  arc A87 (19.76, -23.971051) -> (23.520345, -30.125) centre (65.9053, 0) ccw
  line L109 (59.76, -42.079676) -> (59.76, 37.314927)
  line L110 (59.76, 37.314927) -> (64.76, 33.256172)
  line L111 (64.76, 33.256172) -> (64.76, -29.219299)
  line L112 (64.76, -29.219299) -> (59.76, -42.079676)
  line L113 (108.16, -34.125) -> (112.36, -34.125)
  arc A88 (112.76, -34.525) -> (112.36, -34.125) centre (112.36, -34.525) ccw
  line L114 (112.76, -34.525) -> (112.76, -53.725)
  arc A89 (112.36, -54.125) -> (112.76, -53.725) centre (112.36, -53.725) ccw
  line L115 (112.36, -54.125) -> (108.16, -54.125)
  arc A90 (107.76, -53.725) -> (108.16, -54.125) centre (108.16, -53.725) ccw
  line L116 (107.76, -53.725) -> (107.76, -34.525)
  arc A91 (108.16, -34.125) -> (107.76, -34.525) centre (108.16, -34.525) ccw
  arc A92 (43.76, -39.173788) -> (48.76, -41.605753) centre (65.9053, 0) ccw
  line L117 (43.76, -39.173788) -> (43.76, 39.173788)
  arc A93 (48.76, 41.605753) -> (43.76, 39.173788) centre (65.9053, 0) ccw
  line L118 (48.76, 41.605753) -> (48.76, -41.605753)
  line L119 (51.76, 50.03909) -> (51.76, 53.725)
  arc A94 (52.16, 54.125) -> (51.76, 53.725) centre (52.16, 53.725) ccw
  line L120 (52.16, 54.125) -> (56.36, 54.125)
  arc A95 (56.76, 53.725) -> (56.36, 54.125) centre (56.36, 53.725) ccw
  line L121 (56.76, 53.725) -> (56.76, 51.189486)
  arc A96 (56.76, 51.189486) -> (51.76, 50.03909) centre (65.9053, 0) ccw
  line L122 (48.76, -49.092145) -> (48.76, -53.725)
  arc A97 (48.36, -54.125) -> (48.76, -53.725) centre (48.36, -53.725) ccw
  line L123 (48.36, -54.125) -> (44.16, -54.125)
  arc A98 (43.76, -53.725) -> (44.16, -54.125) centre (44.16, -53.725) ccw
  line L124 (43.76, -53.725) -> (43.76, -47.048759)
  arc A99 (43.76, -47.048759) -> (48.76, -49.092145) centre (65.9053, 0) ccw
  line L125 (51.76, -42.718971) -> (51.76, 42.718971)
  arc A100 (52.72419, 43.026252) -> (51.76, 42.718971) centre (65.9053, 0) ccw
  line L126 (52.72419, 43.026252) -> (56.76, 39.750179)
  line L127 (56.76, 39.750179) -> (56.76, -44.060907)
  arc A101 (51.76, -42.718971) -> (56.76, -44.060907) centre (65.9053, 0) ccw
  line L128 (24.76, 34.125) -> (20.16, 34.125)
  arc A102 (19.76, 34.525) -> (20.16, 34.125) centre (20.16, 34.525) ccw
  line L129 (19.76, 34.525) -> (19.76, 53.725)
  arc A103 (20.16, 54.125) -> (19.76, 53.725) centre (20.16, 53.725) ccw
  line L130 (20.16, 54.125) -> (24.36, 54.125)
  arc A104 (24.76, 53.725) -> (24.36, 54.125) centre (24.36, 53.725) ccw
  line L131 (24.76, 53.725) -> (24.76, 34.125)
  line L132 (72.76, -27.960124) -> (72.76, -44.474859)
  arc A105 (67.76, -44.961763) -> (72.76, -44.474859) centre (65.9053, 0) ccw
  line L133 (67.76, -44.961763) -> (67.76, -40.820501)
  line L134 (67.76, -40.820501) -> (72.76, -27.960124)
  line L135 (75.76, -0.926469) -> (75.76, 24.326911)
  line L136 (75.76, 24.326911) -> (80.76, 20.268157)
  line L137 (80.76, 20.268157) -> (80.76, 11.933908)
  line L138 (80.76, 11.933908) -> (75.76, -0.926469)
  line L139 (104.76, -10.639235) -> (104.76, -22.700491)
  arc A106 (99.76, -29.645561) -> (104.76, -22.700491) centre (65.9053, 0) ccw
  line L140 (99.76, -29.645561) -> (99.76, -12.826549)
  line L141 (99.76, -12.826549) -> (104.76, -10.639235)
  line L142 (107.76, -1.686342) -> (107.76, 16.528281)
  arc A107 (110.904226, -0.31086) -> (107.76, 16.528281) centre (65.9053, 0) ccw
  line L143 (110.904226, -0.31086) -> (107.76, -1.686342)
  line L144 (91.76, -8.685747) -> (91.76, 20.90931)
  line L145 (91.76, 20.90931) -> (96.47099, 33.026332)
  arc A108 (96.76, 32.756488) -> (96.47099, 33.026332) centre (65.9053, 0) ccw
  line L146 (96.76, 32.756488) -> (96.76, -6.498433)
  line L147 (96.76, -6.498433) -> (91.76, -8.685747)
  line L148 (80.76, -21.138342) -> (80.76, -42.477499)
  arc A109 (75.76, -43.907686) -> (80.76, -42.477499) centre (65.9053, 0) ccw
  line L149 (75.76, -43.907686) -> (75.76, -23.325656)
  line L150 (75.76, -23.325656) -> (80.76, -21.138342)
  line L151 (83.76, -12.185449) -> (83.76, 0.332706)
  line L152 (83.76, 0.332706) -> (88.76, 13.193084)
  line L153 (88.76, 13.193084) -> (88.76, -9.998135)
  line L154 (88.76, -9.998135) -> (83.76, -12.185449)
  line L155 (115.76, 34.525) -> (115.76, 53.725)
  arc A110 (116.16, 54.125) -> (115.76, 53.725) centre (116.16, 53.725) ccw
  line L156 (116.16, 54.125) -> (120.36, 54.125)
  arc A111 (120.76, 53.725) -> (120.36, 54.125) centre (120.36, 53.725) ccw
  line L157 (120.76, 53.725) -> (120.76, 34.525)
  arc A112 (120.36, 34.125) -> (120.76, 34.525) centre (120.36, 34.525) ccw
  line L158 (120.36, 34.125) -> (116.16, 34.125)
  arc A113 (115.76, 34.525) -> (116.16, 34.125) centre (116.16, 34.525) ccw
  line L159 (8.36, 34.125) -> (5.4, 34.125)
  arc A114 (5, 34.525) -> (5.4, 34.125) centre (5.4, 34.525) ccw
  line L160 (5, 34.525) -> (5, 47.125)
  arc A115 (8.139394, 52.964154) -> (5, 47.125) centre (12, 47.125) ccw
  arc A116 (8.76, 52.630488) -> (8.139394, 52.964154) centre (8.36, 52.630488) ccw
  line L161 (8.76, 52.630488) -> (8.76, 34.525)
  arc A117 (8.36, 34.125) -> (8.76, 34.525) centre (8.36, 34.525) ccw
  line L162 (16.36, 34.125) -> (12.16, 34.125)
  arc A118 (11.76, 34.525) -> (12.16, 34.125) centre (12.16, 34.525) ccw
  line L163 (11.76, 34.525) -> (11.76, 53.725)
  arc A119 (12.16, 54.125) -> (11.76, 53.725) centre (12.16, 53.725) ccw
  line L164 (12.16, 54.125) -> (16.36, 54.125)
  arc A120 (16.76, 53.725) -> (16.36, 54.125) centre (16.36, 53.725) ccw
  line L165 (16.76, 53.725) -> (16.76, 34.525)
  arc A121 (16.36, 34.125) -> (16.76, 34.525) centre (16.36, 34.525) ccw
  line L166 (128.76, -34.525) -> (128.76, -53.725)
  arc A122 (128.36, -54.125) -> (128.76, -53.725) centre (128.36, -53.725) ccw
  line L167 (128.36, -54.125) -> (124.16, -54.125)
  arc A123 (123.76, -53.725) -> (124.16, -54.125) centre (124.16, -53.725) ccw
  line L168 (123.76, -53.725) -> (123.76, -34.525)
  arc A124 (124.16, -34.125) -> (123.76, -34.525) centre (124.16, -34.525) ccw
  line L169 (124.16, -34.125) -> (128.36, -34.125)
  arc A125 (128.76, -34.525) -> (128.36, -34.125) centre (128.36, -34.525) ccw
  arc A126 (108.290254, -30.125) -> (112.76, -22.552984) centre (65.9053, 0) ccw
  line L170 (112.76, -22.552984) -> (112.76, -29.725)
  arc A127 (112.36, -30.125) -> (112.76, -29.725) centre (112.36, -29.725) ccw
  line L171 (112.36, -30.125) -> (108.290254, -30.125)
  line L172 (107.76, 34.525) -> (107.76, 53.725)
  arc A128 (108.16, 54.125) -> (107.76, 53.725) centre (108.16, 53.725) ccw
  line L173 (108.16, 54.125) -> (112.36, 54.125)
  arc A129 (112.76, 53.725) -> (112.36, 54.125) centre (112.36, 53.725) ccw
  line L174 (112.76, 53.725) -> (112.76, 34.525)
  arc A130 (112.36, 34.125) -> (112.76, 34.525) centre (112.36, 34.525) ccw
  line L175 (112.36, 34.125) -> (108.16, 34.125)
  arc A131 (107.76, 34.525) -> (108.16, 34.125) centre (108.16, 34.525) ccw
  arc A132 (23.520345, 30.125) -> (19.76, 23.971051) centre (65.9053, 0) ccw
  line L176 (19.76, 23.971051) -> (19.76, 29.725)
  arc A133 (20.16, 30.125) -> (19.76, 29.725) centre (20.16, 29.725) ccw
  line L177 (20.16, 30.125) -> (23.520345, 30.125)
  line L178 (24.76, -34.525) -> (24.76, -53.725)
  arc A134 (24.36, -54.125) -> (24.76, -53.725) centre (24.36, -53.725) ccw
  line L179 (24.36, -54.125) -> (20.16, -54.125)
  arc A135 (19.76, -53.725) -> (20.16, -54.125) centre (20.16, -53.725) ccw
  line L180 (19.76, -53.725) -> (19.76, -34.525)
  arc A136 (20.16, -34.125) -> (19.76, -34.525) centre (20.16, -34.525) ccw
  line L181 (20.16, -34.125) -> (24.36, -34.125)
  arc A137 (24.76, -34.525) -> (24.36, -34.125) centre (24.36, -34.525) ccw
  line L182 (132.16, -34.125) -> (135.12, -34.125)